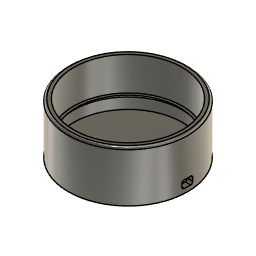
Container v14 (Autodesk Fusion 360 design; units mm, degrees)
Autodesk Fusion 360 part; units mm, degrees
ref_plane "WorkPlane3" through (50, 0, 0) normal (1, 0, 0) x (0, 1, 0) in component "Container"
sketch "Sketch6" plane through (0, 0, 0) normal (0, 1, 0) x (1, 0, 0) in component "Container"
  line L0 (0, 0) -> (55.25, 0)
  line L1 (55.25, 0) -> (55.25, -3)
  line L2 (55.25, -3) -> (0, -3)
  line L3 (0, -3) -> (0, 0)
  line L4 (50.25, -13) -> (55.25, -13)
  line L5 (55.25, -13) -> (55.25, -3)
  line L6 (55.25, -3) -> (50.25, -3)
  line L7 (50.25, -3) -> (50.25, -13)
  line L8 (50.25, -13) -> (104.5, -13) construction
  line L9 (50.25, -13) -> (47.7874, -16.152)
  line L10 (50.25, -13) -> (104.5, -13) construction
  line L11 (47.7874, -16.152) -> (55.25, -16.152)
  line L12 (55.25, -13) -> (55.25, -16.152)
  line L13 (50.25, -13) -> (50.25, -16.152) construction
  line L14 (50.25, -16.152) -> (55.25, -16.152)
  line L15 (55.25, -16.152) -> (55.25, -47.152)
  line L16 (55.25, -47.152) -> (50.25, -47.152)
  line L17 (50.25, -47.152) -> (50.25, -16.152)
  dimension "d44" = 55.25
  dimension "d45" = 3
  dimension "d47" = 10
  dimension "d48" = 10
  dimension "d49" = 5
  dimension "d50" = 5
  dimension "d53" = 128
  dimension "d54" = 4
  dimension "d56" = 3.152
  dimension "d57" = 5
  dimension "d58" = 31
  constraint horizontal L0
  constraint vertical L1
  constraint horizontal L2
  constraint vertical L3
  constraint coincident L0.start L3.end
  constraint horizontal L4
  constraint vertical L5
  constraint horizontal L6
  constraint vertical L7
  constraint horizontal L8
  constraint horizontal L10
  constraint perpendicular L11 L12
  constraint coincident L11 L13.end
  constraint perpendicular L11 L13
  constraint horizontal L14
  constraint vertical L15
  constraint horizontal L16
  constraint vertical L17
  measures "d44" distance of L0.start L0.end
  measures "d45" distance of L0.start L2.end
  measures "d47" distance of L4 L6
  measures "d48" distance of L2 L4
  measures "d49" distance of L5 L7
  measures "d50" distance of L1 L7
  measures "d53" angle of L9 L10
  measures "d54" distance of L4.start L9.end
  measures "d56" distance of L4.end L11.end
  measures "d57" distance of L15 L17
  measures "d58" distance of L11 L16
revolve "Revolve1" add sketch "Sketch6" angle 360 about axis through (0, 0, 1.75) along (0, 0, 1) makes body 1 in component "Container"
fillet "Fillet2" radius 2 1 edges at (-51.5111, -19.9793, 47.152) on bodies 1 in component "Container"
copy_body "CutPasteBodies1" bodies 1 removing the originals makes body 2 in component "Container"
sketch "Sketch8" plane through (50, 0, 0) normal (1, 0, 0) x (0, 1, 0)
  line L0 (-5, 11) -> (5, 11)
  line L1 (5, 11) -> (5, 4)
  line L2 (5, 4) -> (-5, 4)
  line L3 (-5, 4) -> (-5, 11)
  dimension "d71" = 7
  dimension "d72" = 10
  dimension "d73" = 5
  dimension "d74" = 4
  constraint horizontal L0
  constraint vertical L1
  constraint horizontal L2
  constraint vertical L3
  measures "d71" distance of L0 L2
  measures "d72" distance of L1 L3
  measures "d73" distance of origin L1
  measures "d74" distance of origin L2
extrude "Extrude1" cut sketch "Sketch8" along normal blind 17 bodies 2 in component "Container"
fillet "Fillet1" radius 2 4 edges at (52.512, -5, 11) (52.512, 5, 11) (52.512, -5, 4) (52.512, 5, 4) on bodies 2 in component "Container"
component "Container" placed x (1, 0, 0) y (0, 1, 0) z (0, 0, 1) at (0, 0, 0)
equation "d44 = ( 100.5 / 2 ) * 1 mm + d49"
equation "d48 = d47"
equation "d50 = d49"
equation "d53 = 90 deg + 38 deg"
equation "d57 = d49"
equation "d73 = d72 / 2"
equation "d74 = 3.00 mm + 1 mm"
